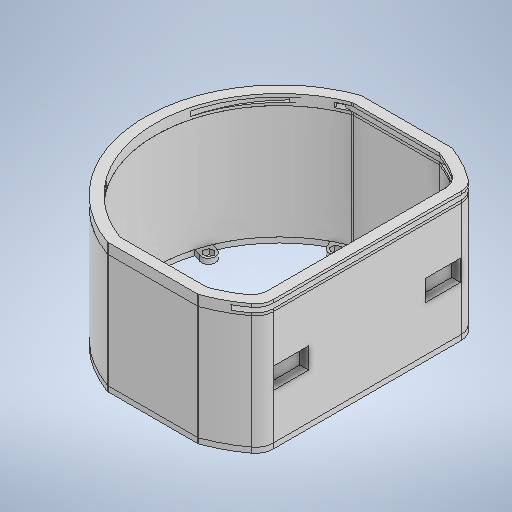
# Autodesk Inventor part: carcasa4.0
Saved by Autodesk Inventor 2025.3 (Build 293356030, 356C)
## iProperties
Created: 2025-08-27
Part Number: carcasa4.0
Material: Generic
Document SubType Name: Modeling
Designer: cdavi
Density: 1 g/cm^3
Appearance: Default
Author: cdavi
Autodesk Inventor part; units mm, degrees
ref_plane "YZ Plane" through (0, 0, 0) normal (1, 0, 0) x (0, 1, 0)
ref_plane "XZ Plane" through (0, 0, 0) normal (0, 1, 0) x (-1, 0, 0)
ref_plane "XY Plane" through (0, 0, 0) normal (0, 0, 1) x (1, 0, 0)
sketch "Sketch1" plane through (0, 0, 0) normal (0, 1, 0) x (-1, 0, 0)
  line L0 (24.5102, 66.5) -> (-24.5102, 66.5)
  line L1 (0, 0) -> (-50, 0) construction
  line L2 (25.5881, 72.5) -> (-25.5881, 72.5)
  line L3 (24.5102, -66.5) -> (-24.8747, -66.5)
  line L4 (25.5881, -72.5) -> (-25.5881, -72.5)
  line L5 (0, 0) -> (0, 72.5) construction
  line L6 (-44, 50.6458) -> (-44, -50.6458)
  line L7 (-50, 53.7494) -> (-50, -53.7494)
  arc A0 (-39.5738, -58.9484) -> (-24.8747, -66.5) centre (0, 0) ccw
  arc A1 (-45.9701, -61.7717) -> (-26.2704, -72.38) centre (0, 0) ccw
  arc A2 (26.2704, -72.38) -> (26.2704, 72.38) centre (0, 0) ccw
  arc A3 (-26.2704, 72.38) -> (-45.9701, 61.7717) centre (0, 0) ccw
  arc A4 (25.2206, -66.3696) -> (25.2206, 66.3696) centre (0, 0) ccw
  arc A5 (-25.2206, 66.3696) -> (-39.5738, 58.9484) centre (0, 0) ccw
  arc A6 (-26.2704, -72.38) -> (-25.5881, -72.5) centre (-25.5881, -70.5) ccw
  arc A7 (25.5881, -72.5) -> (26.2704, -72.38) centre (25.5881, -70.5) ccw
  arc A8 (24.5102, -66.5) -> (25.2206, -66.3696) centre (24.5102, -64.5) ccw
  arc A9 (25.2206, 66.3696) -> (24.5102, 66.5) centre (24.5102, 64.5) ccw
  arc A10 (26.2704, 72.38) -> (25.5881, 72.5) centre (25.5881, 70.5) ccw
  arc A11 (-24.5102, 66.5) -> (-25.2206, 66.3696) centre (-24.5102, 64.5) ccw
  arc A12 (-25.5881, 72.5) -> (-26.2704, 72.38) centre (-25.5881, 70.5) ccw
  arc A13 (-39.5738, 58.9484) -> (-44, 50.6458) centre (-34, 50.6458) ccw
  arc A14 (-45.9701, 61.7717) -> (-50, 53.7494) centre (-40, 53.7494) ccw
  arc A15 (-50, -53.7494) -> (-45.9701, -61.7717) centre (-40, -53.7494) ccw
  arc A16 (-44, -50.6458) -> (-39.5738, -58.9484) centre (-34, -50.6458) ccw
  point P0 (-25.9374, 72.5)
  point P1 (24.8747, -66.5)
  point P2 (25.9374, -72.5)
  point P3 (-25.9374, -72.5)
  point P4 (-50, -58.5577)
  point P5 (-44, 55.7225)
  point P6 (-44, -55.7225)
  point P7 (-50, 58.5577)
  point P8 (25.9374, 72.5)
  point P9 (24.8747, 66.5)
  point P10 (-24.8747, 66.5)
  dimension "d2" = 66.5
  dimension "d4" = 6
  dimension "d6" = 44
  dimension "d7" = 6
  dimension "d8" = 2
  dimension "d9" = 10
  dimension "d10" = 71
  dimension "d11" = 77
  dimension "d12" = 71
  dimension "d13" = 77
  constraints: 45 point on circle, 22 tangent, 17 centre point, 16 end point, 11 point on line, 9 equal radius, 4 symmetric about line, 3 vertical, 2 coincident, 2 horizontal, 2 midpoint, 1 parallel
  measures "d2" distance between parallel lines of L1 L0
  measures "d4" distance between parallel lines of L0 L2
  measures "d6" distance between parallel lines of L6 L5
  measures "d7" distance between parallel lines of L7 L6
  measures "d8" radius of A6
  measures "d9" radius of A13
  measures "d10" radius of A4
  measures "d11" radius of A2
  measures "d12" radius of A0
  measures "d13" radius of A1
extrude "Extrusion1" add sketch "Sketch1" along normal blind 65
sketch "Sketch2" plane through (50, 0, 53.7494) normal (1, 0, 0) x (0, 0, -1)
  line L0 (53.7494, 0) -> (53.7494, 65) construction
  line L1 (104.3952, 65) -> (3.1036, 65) projected
  line L2 (0.3694, 38) -> (20.3694, 38)
  line L3 (20.3694, 38) -> (20.3694, 26)
  line L4 (20.3694, 26) -> (0.3694, 26)
  line L5 (0.3694, 26) -> (0.3694, 38)
  line L6 (0, 0) -> (107.4988, 0) projected
  line L7 (-18.6306, 0) -> (-18.6306, 65) projected
  line L8 (107.1294, 38) -> (87.1294, 38)
  line L9 (87.1294, 38) -> (87.1294, 26)
  line L10 (87.1294, 26) -> (107.1294, 26)
  line L11 (107.1294, 26) -> (107.1294, 38)
  dimension "d16" = 26
  dimension "d17" = 19
  dimension "d18" = 12
  dimension "d19" = 20
  constraints: 18 end point, 4 symmetric about line, 2 parallel, 1 horizontal, 1 midpoint, 1 perpendicular
  measures "d16" distance between parallel lines of L6 L4
  measures "d17" distance between parallel lines of L5 L7
  measures "d18" distance of L2.end L3.end
  measures "d19" distance of L2.start L2.end
extrude "Extrusion2" cut sketch "Sketch2" against normal blind 5
sketch "Sketch3" plane through (50, 0, 53.7494) normal (1, 0, 0) x (0, 0, -1)
  line L0 (3.568, 49.2223) -> (17.7975, 43.9952) construction
  line L1 (2.8909, 47.379) -> (17.1204, 42.1519)
  line L2 (18.4746, 45.8385) -> (4.2452, 51.0656)
  arc A0 (4.2452, 51.0656) -> (2.8909, 47.379) centre (3.568, 49.2223) ccw
  arc A1 (17.1204, 42.1519) -> (18.4746, 45.8385) centre (17.7975, 43.9952) ccw
  arc A2 (44.4296, 11.624) -> (34.6921, 2.9774) centre (43.8866, 2.4292) ccw construction
  arc A3 (44.531, 13.3402) -> (32.9759, 3.0797) centre (43.8866, 2.4292) ccw
  arc A4 (44.3283, 9.9077) -> (36.4083, 2.8751) centre (43.8866, 2.4292) ccw
  arc A5 (44.3283, 9.9077) -> (44.531, 13.3402) centre (44.4296, 11.624) ccw
  arc A6 (32.9759, 3.0797) -> (36.4083, 2.8751) centre (34.6921, 2.9774) ccw
  line L3 (53.7494, 0) -> (53.7494, 65) construction
  line L4 (104.6079, 47.379) -> (90.3785, 42.1519)
  line L5 (89.0242, 45.8385) -> (103.2537, 51.0656)
  arc A7 (104.6079, 47.379) -> (103.2537, 51.0656) centre (103.9308, 49.2223) ccw
  arc A8 (89.0242, 45.8385) -> (90.3785, 42.1519) centre (89.7013, 43.9952) ccw
  point P0 (10.6828, 46.6088)
  constraints: 18 point on circle, 12 end point, 9 centre point, 8 tangent, 6 symmetric about line, 1 midpoint, 1 parallel, 2 other
extrude "Extrusion3" [suppressed]
extrude "Extrusion4" add sketch "Sketch1" along normal blind 3 from surface at 65 separate body contours A9 A4 A8 L3 A0 A16 L6 A13 A5 A11 L0 | A10 A2 A7 L4 A6 A1 A15 L7 A14 A3 A12 L2
sketch "Sketch5" plane through (-25.5881, 68, 72.5) normal (0, 1, 0) x (1, 0, 0)
  circle A0 centre (25.5881, 72.5) radius 8.5
  circle A1 centre (-4.4119, 72.5) radius 2.5
  line L0 (33.7121, 70) -> (42.5881, 70)
  line L1 (42.5881, 70) -> (42.5881, 75)
  line L2 (42.5881, 75) -> (33.7121, 75)
  point P0 (42.5881, 72.5)
  dimension "d26" = 17
  dimension "d27" = 5
  dimension "d31" = 5
  dimension "d32" = 17
  dimension "d47" = 30
  constraints: 6 end point, 2 centre point, 2 horizontal alignment, 2 perpendicular, 2 point on circle, 1 coincident, 1 horizontal, 1 midpoint
  measures "d26" diameter of A0
  measures "d27" diameter of A1
  measures "d31" distance between parallel lines of L2 L0
  measures "d32" distance from line of A0.centre L1
  measures "d47" distance of A0.centre A1.centre
extrude "Extrusion5" cut sketch "Sketch5" against normal through all bodies 2
sketch "Sketch6" plane through (0, 0, 0) normal (0, 1, 0) x (-1, 0, 0)
  circle A0 centre (0, 0) radius 66.5 construction
  arc A1 (-25.2206, 66.3696) -> (-39.5738, 58.9484) centre (0, 0) ccw projected
  arc A2 (-39.5738, 58.9484) -> (-44, 50.6458) centre (-34, 50.6458) ccw projected
  line L0 (-44, -50.6458) -> (-44, 50.6458) projected
  arc A3 (-44, -50.6458) -> (-39.5738, -58.9484) centre (-34, -50.6458) ccw projected
  arc A4 (-39.5738, -58.9484) -> (-24.8747, -66.5) centre (0, 0) ccw projected
  line L1 (24.5102, -66.5) -> (-24.8747, -66.5) construction
  arc A5 (25.2206, -66.3696) -> (25.2206, 66.3696) centre (0, 0) ccw projected
  line L2 (-24.5102, 66.5) -> (24.5102, 66.5) construction
  line L3 (25.5881, 72.5) -> (-25.5881, 72.5) projected
  arc A6 (-26.2704, 72.38) -> (-45.9701, 61.7717) centre (0, 0) ccw projected
  arc A7 (-45.9701, 61.7717) -> (-50, 53.7494) centre (-40, 53.7494) ccw projected
  line L4 (-50, 53.7494) -> (-50, -53.7494) projected
  arc A8 (-50, -53.7494) -> (-45.9701, -61.7717) centre (-40, -53.7494) ccw projected
  arc A9 (-45.9701, -61.7717) -> (-26.2704, -72.38) centre (0, 0) ccw projected
  line L5 (-25.5881, -72.5) -> (25.5881, -72.5) projected
  arc A10 (26.2704, -72.38) -> (26.2704, 72.38) centre (0, 0) ccw projected
  arc A11 (-24.125, 60.3571) -> (-36.2295, 53.9669) centre (0, 0) ccw construction
  arc A12 (-36.2295, 53.9669) -> (-38, 50.6458) centre (-34, 50.6458) ccw construction
  line L6 (-38, 50.6458) -> (-38, -50.6458) construction
  arc A13 (-38, -50.6458) -> (-36.2295, -53.9669) centre (-34, -50.6458) ccw construction
  arc A14 (-36.2295, -53.9669) -> (-24.125, -60.3571) centre (0, 0) ccw construction
  line L7 (-23.3827, -60.5) -> (23.3827, -60.5) construction
  line L8 (-23.3827, 60.5) -> (23.3827, 60.5) construction
  arc A15 (24.125, -60.3571) -> (24.125, 60.3571) centre (0, 0) ccw construction
  arc A16 (-8.124, -2.5) -> (-8.124, 2.5) centre (0, 0) ccw projected
  line L9 (0, 0) -> (62.7203, 22.1) construction
  line L10 (0, 0) -> (77, 0) construction
  circle A17 centre (62.7203, 22.1) radius 2.85 construction
  line L11 (0, 0) -> (0, -66.5) construction
  circle A18 centre (28.1041, 60.2695) radius 2.85 construction
  line L12 (28.1041, 60.2695) -> (0, 0) construction
  circle A19 centre (-40.5, 20) radius 2.85 construction
  circle A20 centre (-28.1041, 60.2695) radius 2.85 construction
  line L13 (-28.1041, 60.2695) -> (0, 0) construction
  arc A21 (-23.3827, 60.5) -> (-24.125, 60.3571) centre (-23.3827, 58.5) ccw construction
  arc A22 (-24.125, -60.3571) -> (-23.3827, -60.5) centre (-23.3827, -58.5) ccw construction
  arc A23 (23.3827, -60.5) -> (24.125, -60.3571) centre (23.3827, -58.5) ccw construction
  arc A24 (24.125, 60.3571) -> (23.3827, 60.5) centre (23.3827, 58.5) ccw construction
  arc A25 (-26.2704, -72.38) -> (-25.5881, -72.5) centre (-25.5881, -70.5) ccw projected
  arc A26 (25.5881, -72.5) -> (26.2704, -72.38) centre (25.5881, -70.5) ccw projected
  arc A27 (26.2704, 72.38) -> (25.5881, 72.5) centre (25.5881, 70.5) ccw projected
  arc A28 (-25.5881, 72.5) -> (-26.2704, 72.38) centre (-25.5881, 70.5) ccw projected
  circle A29 centre (62.7203, -22.1) radius 2.85 construction
  circle A30 centre (28.1041, -60.2695) radius 2.85 construction
  circle A31 centre (-40.5, -20) radius 2.85 construction
  circle A32 centre (-28.1041, -60.2695) radius 2.85 construction
  line L14 (25.2206, 59.9076) -> (25.2206, 66.3696)
  line L15 (-25.2206, 59.9076) -> (-25.2206, 66.3696)
  line L16 (25.2206, 66.3696) -> (-25.2206, 66.3696)
  line L17 (25.2206, -59.9076) -> (25.2206, -66.3696)
  line L18 (-25.2206, -59.9076) -> (-25.2206, -66.3696)
  line L19 (25.2206, -66.3696) -> (-25.2206, -66.3696)
  circle A33 centre (62.7203, 22.1) radius 4
  circle A34 centre (28.1041, 60.2695) radius 4
  line L20 (59.9189, 22.6238) -> (61.7732, 24.788)
  line L21 (61.7732, 24.788) -> (64.5746, 24.2643)
  line L22 (64.5746, 24.2643) -> (65.5218, 21.5762)
  line L23 (65.5218, 21.5762) -> (63.6675, 19.412)
  line L24 (63.6675, 19.412) -> (60.866, 19.9357)
  line L25 (60.866, 19.9357) -> (59.9189, 22.6238)
  line L26 (25.7695, 58.6348) -> (25.5211, 61.4739)
  line L27 (25.5211, 61.4739) -> (27.8557, 63.1086)
  line L28 (27.8557, 63.1086) -> (30.4387, 61.9042)
  line L29 (30.4387, 61.9042) -> (30.6871, 59.065)
  line L30 (30.6871, 59.065) -> (28.3525, 57.4303)
  line L31 (28.3525, 57.4303) -> (25.7695, 58.6348)
  circle A35 centre (-40.5, 20) radius 4
  line L32 (-42.9682, 18.575) -> (-42.9682, 21.425)
  line L33 (-42.9682, 21.425) -> (-40.5, 22.85)
  line L34 (-40.5, 22.85) -> (-38.0318, 21.425)
  line L35 (-38.0318, 21.425) -> (-38.0318, 18.575)
  line L36 (-38.0318, 18.575) -> (-40.5, 17.15)
  line L37 (-40.5, 17.15) -> (-42.9682, 18.575)
  line L38 (-40.5, 24) -> (-44, 24)
  line L39 (-40.5, 16) -> (-44, 16)
  circle A36 centre (-28.1041, 60.2695) radius 4
  line L40 (-28.3525, 57.4303) -> (-30.6871, 59.065)
  line L41 (-30.6871, 59.065) -> (-30.4387, 61.9042)
  line L42 (-30.4387, 61.9042) -> (-27.8557, 63.1086)
  line L43 (-27.8557, 63.1086) -> (-25.5211, 61.4739)
  line L44 (-25.5211, 61.4739) -> (-25.7695, 58.6348)
  line L45 (-25.7695, 58.6348) -> (-28.3525, 57.4303)
  line L46 (-31.6769, 58.4707) -> (-33.7013, 62.4918)
  circle A37 centre (62.7203, -22.1) radius 4
  circle A38 centre (28.1041, -60.2695) radius 4
  circle A39 centre (-40.5, -20) radius 4
  line L47 (-40.5, -24) -> (-44, -24)
  line L48 (-40.5, -16) -> (-44, -16)
  circle A40 centre (-28.1041, -60.2695) radius 4
  line L49 (-31.6769, -58.4707) -> (-33.7013, -62.4918)
  line L50 (59.9189, -22.6238) -> (61.7732, -24.788)
  line L51 (61.7732, -24.788) -> (64.5746, -24.2643)
  line L52 (64.5746, -24.2643) -> (65.5218, -21.5762)
  line L53 (65.5218, -21.5762) -> (63.6675, -19.412)
  line L54 (63.6675, -19.412) -> (60.866, -19.9357)
  line L55 (60.866, -19.9357) -> (59.9189, -22.6238)
  line L56 (25.7695, -58.6348) -> (25.5211, -61.4739)
  line L57 (25.5211, -61.4739) -> (27.8557, -63.1086)
  line L58 (27.8557, -63.1086) -> (30.4387, -61.9042)
  line L59 (30.4387, -61.9042) -> (30.6871, -59.065)
  line L60 (30.6871, -59.065) -> (28.3525, -57.4303)
  line L61 (28.3525, -57.4303) -> (25.7695, -58.6348)
  line L62 (-28.3525, -57.4303) -> (-30.6871, -59.065)
  line L63 (-30.6871, -59.065) -> (-30.4387, -61.9042)
  line L64 (-30.4387, -61.9042) -> (-27.8557, -63.1086)
  line L65 (-27.8557, -63.1086) -> (-25.5211, -61.4739)
  line L66 (-25.5211, -61.4739) -> (-25.7695, -58.6348)
  line L67 (-25.7695, -58.6348) -> (-28.3525, -57.4303)
  line L68 (-42.9682, -18.575) -> (-42.9682, -21.425)
  line L69 (-42.9682, -21.425) -> (-40.5, -22.85)
  line L70 (-40.5, -22.85) -> (-38.0318, -21.425)
  line L71 (-38.0318, -21.425) -> (-38.0318, -18.575)
  line L72 (-38.0318, -18.575) -> (-40.5, -17.15)
  line L73 (-40.5, -17.15) -> (-42.9682, -18.575)
  line L74 (61.2781, 25.831) -> (65.4773, 27.4541)
  line L75 (63.9356, 18.2891) -> (68.2247, 19.6568)
  line L76 (31.6769, 58.4707) -> (33.7013, 62.4918)
  line L77 (61.2781, -25.831) -> (65.4773, -27.4541)
  line L78 (63.9356, -18.2891) -> (68.2247, -19.6568)
  line L79 (31.6769, -58.4707) -> (33.7013, -62.4918)
  line L80 (-24.4297, 61.8501) -> (-26.2087, 65.9856)
  line L81 (24.4297, 61.8501) -> (26.2087, 65.9856)
  line L82 (-24.4297, -61.8501) -> (-26.2087, -65.9856)
  line L83 (24.4297, -61.8501) -> (26.2087, -65.9856)
  line L84 (-24.5102, 66.5) -> (-50, 66.5)
  line L85 (-50, 66.5) -> (-50, 53.7494)
  line L86 (-38.8169, 66.5) -> (-24.5102, 66.5)
  point P0 (-23.7645, -60.5)
  point P1 (-25.2206, 59.9076)
  point P2 (25.2206, -59.9076)
  point P3 (-25.2206, -59.9076)
  point P4 (-25.2206, -66.3696)
  point P5 (-33.7013, -62.4918)
  point P6 (-44, -24)
  point P7 (68.2247, -19.6568)
  point P8 (63.9356, -18.2891)
  point P9 (61.2781, -25.831)
  point P10 (33.7013, -62.4918)
  point P11 (31.6769, -58.4707)
  point P12 (-30.0059, 64.3479)
  point P13 (-30.0059, -64.3479)
  point P14 (26.7854, -65.7536)
  point P15 (26.7854, 65.7536)
  point P16 (-44, 21.9365)
  point P17 (-44, 18.0635)
  point P18 (-33.1529, 62.7844)
  point P19 (30.0059, -64.3479)
  point P20 (66.9646, -23.5955)
  point P21 (65.7151, -26.8798)
  point P22 (-33.1529, -62.7844)
  point P23 (-44, -21.9365)
  point P24 (-44, -18.0635)
  point P25 (65.7151, 26.8798)
  point P26 (66.9646, 23.5955)
  point P27 (30.0059, 64.3479)
  point P28 (24.4297, -61.8501)
  point P29 (26.2087, -65.9856)
  point P30 (-26.2087, -65.9856)
  point P31 (-24.4297, -61.8501)
  point P32 (25.2206, -63.2254)
  point P33 (-26.8685, -67.3194)
  point P34 (26.8685, -67.3194)
  point P35 (26.8685, 67.3194)
  point P36 (-26.8685, 67.3194)
  point P37 (25.2206, 63.2254)
  point P38 (-25.2206, -66.3696)
  point P39 (-25.2206, -63.0418)
  point P40 (-25.2206, 63.0418)
  point P41 (25.2206, 63.0418)
  point P42 (-25.2206, -61.8451)
  point P43 (25.2206, -63.0418)
  point P44 (-25.2206, 61.8451)
  point P45 (25.2206, -63.6888)
  point P46 (-25.2206, -63.6888)
  dimension "d33" = 133
  dimension "d39" = 5.7
  dimension "d34" = 6
  dimension "d35" = 6
  dimension "d36" = 6
  dimension "d37" = 19.41
  dimension "d38" = 25
  dimension "d40" = 20
  dimension "d41" = 3.5
  dimension "d42" = 25
  dimension "d44" = 2
  dimension "d61" = 8
  dimension "d62" = 8
  dimension "d63" = 8
  dimension "d64" = 8
  dimension "d171" = 90
  dimension "d172" = 12.7506
  constraints: 162 end point, 52 symmetric about line, 38 point on circle, 20 centre point, 16 tangent, 10 coincident, 6 perpendicular, 4 point on line, 3 equal radius, 2 parallel, 2 vertical, 1 collinear, 1 horizontal, 93 other
  measures "d34" radial gap between concentric circles of A1 A11
  measures "d35" distance between parallel lines of L2 L8
  measures "d36" radial gap between concentric circles of A5 A15
  measures "d37" angle of L10 L9
  measures "d38" angle of L11 L12
  measures "d40" distance from line of point (-40.5, 20) L10
  measures "d41" distance from line of L0 point (-40.5, 20)
  measures "d42" angle of L11 L13
  measures "d44" radius of A21
  measures "d61" diameter of A33
  measures "d62" diameter of A34
  measures "d63" diameter of A35
  measures "d64" diameter of A36
  measures "d171" angle of L85 L84
  measures "d172" distance of L84.end L4.start
extrude "Extrusion6" add sketch "Sketch6" against normal blind 3 separate body contours L15 L80 A1 | L80 L15 A36 L46 A1 | A36 | A5 L76 A34 L14 L81 | L14 A34 L81 | A34 | A5 L75 A33 L74 | L38 A35 L0 | A33 | A35 L0 | A5 L77 A37 L78 | A35 L39 L0 | A37 | A5 L83 L17 A38 L79 | L48 A39 L0 | A38 | A39 L0 | A39 L47 L0 | A4 L49 A40 L18 L82 | A40 | A27 A10 A26 L5 A25 A9 A8 L4 A7 A6 A28 L3 picked at (-37.5212, 20) picked at (-37.5212, -20)
sketch "Sketch14" plane through (0, 65, 0) normal (0, 1, 0) x (1, 0, 0)
  arc A0 (-26.2704, 72.38) -> (-26.2704, -72.38) centre (0, 0) ccw projected
  arc A1 (-26.2704, -72.38) -> (-25.5881, -72.5) centre (-25.5881, -70.5) ccw projected
  line L0 (-25.5881, -72.5) -> (25.5881, -72.5) projected
  arc A2 (25.5881, -72.5) -> (26.2704, -72.38) centre (25.5881, -70.5) ccw projected
  arc A3 (26.2704, -72.38) -> (45.9701, -61.7717) centre (0, 0) ccw projected
  arc A4 (45.9701, -61.7717) -> (50, -53.7494) centre (40, -53.7494) ccw projected
  line L1 (50, -53.7494) -> (50, 53.7494) projected
  arc A5 (50, 53.7494) -> (45.9701, 61.7717) centre (40, 53.7494) ccw projected
  arc A6 (45.9701, 61.7717) -> (26.2704, 72.38) centre (0, 0) ccw projected
  arc A7 (26.2704, 72.38) -> (25.5881, 72.5) centre (25.5881, 70.5) ccw projected
  line L2 (25.5881, 72.5) -> (-25.5881, 72.5) projected
  arc A8 (-25.5881, 72.5) -> (-26.2704, 72.38) centre (-25.5881, 70.5) ccw projected
  line L3 (-24.5102, 66.5) -> (24.8747, 66.5) projected
  arc A9 (39.5738, 58.9484) -> (24.8747, 66.5) centre (0, 0) ccw projected
  arc A10 (44, 50.6458) -> (39.5738, 58.9484) centre (34, 50.6458) ccw projected
  line L4 (44, 50.6458) -> (44, -50.6458) projected
  arc A11 (39.5738, -58.9484) -> (44, -50.6458) centre (34, -50.6458) ccw projected
  arc A12 (25.2206, -66.3696) -> (39.5738, -58.9484) centre (0, 0) ccw projected
  arc A13 (24.5102, -66.5) -> (25.2206, -66.3696) centre (24.5102, -64.5) ccw projected
  line L5 (24.5102, -66.5) -> (-24.5102, -66.5) projected
  arc A14 (-25.2206, -66.3696) -> (-24.5102, -66.5) centre (-24.5102, -64.5) ccw projected
  arc A15 (-25.2206, 66.3696) -> (-25.2206, -66.3696) centre (0, 0) ccw projected
  arc A16 (-24.5102, 66.5) -> (-25.2206, 66.3696) centre (-24.5102, 64.5) ccw projected
extrude "Extrusion11" add sketch "Sketch14" along normal blind 6 separate body
sketch "Sketch15" plane through (50, 65, 53.7494) normal (1, 0, 0) x (0, 0, -1)
  line L0 (53.7494, 6) -> (53.7494, 0)
  line L1 (53.7494, 6) -> (0, 6)
  line L2 (0, 6) -> (-12.763, 6)
  line L3 (-12.763, 6) -> (-12.763, 0)
  line L4 (-12.763, 0) -> (0, 0)
  line L5 (0, 0) -> (53.7494, 0)
  line L6 (3.1036, 0) -> (53.7494, 0)
  line L7 (53.7494, 6) -> (0, 6)
  line L8 (53.7494, 6) -> (53.7494, 4.5)
  line L9 (53.7494, 4.5) -> (0, 4.246)
  line L10 (0, 0) -> (0, 6) projected
  line L11 (53.7494, 0) -> (53.7494, 1.5)
  line L12 (53.7494, 1.5) -> (0, 1.5)
  arc A0 (53.7494, 4.5) -> (53.7494, 4.5) centre (52.9973, 163.6577) ccw
  line L13 (0, 4.246) -> (-12.763, 4.246)
  line L14 (0, 1.5) -> (-12.763, 1.5)
  line L15 (53.7494, 6) -> (107.4988, 6)
  line L16 (107.4988, 6) -> (120.2618, 6)
  line L17 (120.2618, 6) -> (120.2618, 0)
  line L18 (120.2618, 0) -> (107.4988, 0)
  line L19 (107.4988, 0) -> (53.7494, 0)
  line L20 (104.3952, 0) -> (53.7494, 0)
  line L21 (53.7494, 6) -> (107.4988, 6)
  line L22 (53.7494, 4.5) -> (107.4988, 4.246)
  line L23 (107.4988, 0) -> (107.4988, 6)
  line L24 (53.7494, 1.5) -> (107.4988, 1.5)
  arc A1 (53.7494, 4.5) -> (53.7494, 4.5) centre (54.5015, 163.6577) ccw
  line L25 (107.4988, 4.246) -> (120.2618, 4.246)
  line L26 (107.4988, 1.5) -> (120.2618, 1.5)
  point P0 (53.7494, -65)
  dimension "d173" = 12.763
  dimension "d176" = 1.5
  dimension "d177" = 1.5
  dimension "d202" = 2.746
  constraints: 52 end point, 15 point on line, 11 symmetric about line, 6 perpendicular, 4 point on circle, 2 centre point, 1 collinear, 1 tangent, 1 other
  measures "d173" distance of L1.end L2.end
  measures "d176" distance of L0.start L8.end
  measures "d177" distance of L0.end L11.end
  measures "d202" distance between parallel lines of L14 L13
extrude "Extrusion12" cut sketch "Sketch15" against normal blind 82.146 contours L22 L23 L24 L0 | L0 L12 L10 L9 | L10 L14 L3 L13 | L25 L17 L26 L23 bodies 4
ref_plane "Work Plane1" through (0, 66.5, 0) normal (0, -1, 0) x (1, 0, 0)
sketch "Sketch18" plane through (0, 66.5, 0) normal (0, -1, 0) x (1, 0, 0)
  arc A0 (-24.5102, 66.6923) -> (-24.5102, -68.6923) centre (5.3854, -1) ccw
  arc A1 (-24.5102, 68.8731) -> (-24.5102, -70.8731) centre (5.3854, -1) ccw
  line L0 (24.8747, -66.5) -> (-24.5102, -66.5) projected
  line L1 (-24.5102, -66.5) -> (-24.5102, -70.8731)
  line L2 (-24.5102, 66.5) -> (24.5102, 66.5) projected
  line L3 (-24.5102, 66.5) -> (-24.5102, 68.8731)
  point P0 (-25.2206, -66.3696)
  point P1 (-25.2206, 66.3696)
  point P2 (-29.896, -69.4992)
  dimension "d199" = 152
  constraints: 5 end point, 4 point on circle, 2 centre point, 2 coincident, 2 point on line, 1 perpendicular, 1 vertical
  measures "d199" diameter of A1
extrude "Extrusion14" cut sketch "Sketch18" against normal blind 2.746 bodies 4
body "Solid1"
body "Solid2"
body "Solid3"
body "Solid4"
